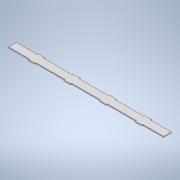
# Autodesk Inventor part: BungaSign-Bigger-Sides-TopBottom
Saved by Autodesk Inventor 2022 (Build 260153000, 153)
## iProperties
Created: 2022-08-22
Part Number: BungaSign-Bigger-Sides-TopBottom
Material: Generic
Document SubType Name: Modeling
Designer: incep
Density: 1 g/cm^3
Appearance: Default
Author: incep
Autodesk Inventor part; units mm, degrees
ref_plane "YZ Plane" through (0, 0, 0) normal (1, 0, 0) x (0, 1, 0)
ref_plane "XZ Plane" through (0, 0, 0) normal (0, 1, 0) x (-1, 0, 0)
ref_plane "XY Plane" through (0, 0, 0) normal (0, 0, 1) x (1, 0, 0)
sketch "Sketch1" plane through (0, 0, 0) normal (0, 1, 0) x (-1, 0, 0)
  line L0 (232, -11.5) -> (-232, -11.5)
  line L1 (-232, -11.5) -> (-232, 11.5)
  line L2 (-232, 11.5) -> (232, 11.5)
  line L3 (232, 11.5) -> (232, -11.5)
  line L4 (170.5, -14.5) -> (150.5, -14.5)
  line L5 (150.5, -14.5) -> (150.5, -11.5)
  line L6 (150.5, -11.5) -> (170.5, -11.5)
  line L7 (170.5, -11.5) -> (170.5, -14.5)
  line L8 (160.5, -14.5) -> (160.5, -11.5)
  line L9 (170.5, 11.5) -> (150.5, 11.5)
  line L10 (150.5, 11.5) -> (150.5, 14.5)
  line L11 (150.5, 14.5) -> (170.5, 14.5)
  line L12 (170.5, 14.5) -> (170.5, 11.5)
  line L13 (63.5, -14.5) -> (43.5, -14.5)
  line L14 (43.5, -14.5) -> (43.5, -11.5)
  line L15 (43.5, -11.5) -> (63.5, -11.5)
  line L16 (63.5, -11.5) -> (63.5, -14.5)
  line L17 (53.5, -14.5) -> (53.5, -11.5)
  line L18 (63.5, 11.5) -> (43.5, 11.5)
  line L19 (43.5, 11.5) -> (43.5, 14.5)
  line L20 (43.5, 14.5) -> (63.5, 14.5)
  line L21 (63.5, 14.5) -> (63.5, 11.5)
  line L22 (-43.5, -14.5) -> (-63.5, -14.5)
  line L23 (-63.5, -14.5) -> (-63.5, -11.5)
  line L24 (-63.5, -11.5) -> (-43.5, -11.5)
  line L25 (-43.5, -11.5) -> (-43.5, -14.5)
  line L26 (-53.5, -14.5) -> (-53.5, -11.5)
  line L27 (-43.5, 11.5) -> (-63.5, 11.5)
  line L28 (-63.5, 11.5) -> (-63.5, 14.5)
  line L29 (-63.5, 14.5) -> (-43.5, 14.5)
  line L30 (-43.5, 14.5) -> (-43.5, 11.5)
  line L31 (-150.5, -14.5) -> (-170.5, -14.5)
  line L32 (-170.5, -14.5) -> (-170.5, -11.5)
  line L33 (-170.5, -11.5) -> (-150.5, -11.5)
  line L34 (-150.5, -11.5) -> (-150.5, -14.5)
  line L35 (-160.5, -14.5) -> (-160.5, -11.5)
  line L36 (-150.5, 11.5) -> (-170.5, 11.5)
  line L37 (-170.5, 11.5) -> (-170.5, 14.5)
  line L38 (-170.5, 14.5) -> (-150.5, 14.5)
  line L39 (-150.5, 14.5) -> (-150.5, 11.5)
  point P0 (0, 0)
  point P1 (-232, 0)
  point P2 (0, -11.5)
  dimension "d0" = 464
  dimension "d1" = 23
  dimension "d2" = 3
  dimension "d3" = 20
  dimension "d4" = 160.5
  dimension "d5" = 3
  dimension "d9" = 107
  dimension "d14" = 20
  constraints: 80 end point, 6 parallel, 4 collinear, 4 horizontal, 4 midpoint, 3 perpendicular, 1 horizontal alignment, 1 vertical alignment, 56 other
  measures "d0" distance of L0.start L0.end
  measures "d1" distance of L2.end L0.start
  measures "d2" distance of L4.end L5.end
  measures "d3" distance of L4.start L4.end
  measures "d4" horizontal distance of point (0, 0) L8.start
  measures "d5" distance of L9.end L10.end
  measures "d9" distance of L4.start L13.start
  measures "d14" distance of L10.end L11.end
extrude "Extrusion1" add sketch "Sketch1" along normal blind 3
equation "\"d1\" = stack"
equation "\"d2\" = thickness"
equation "\"d3\" = finger"
equation "\"d5\" = thickness"
equation "\"d14\" = finger"
equation "\"stack\" = 23"
equation "\"thickness\" = 3"
equation "\"finger\" = 20"
body "Solid1"
